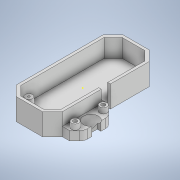
# Autodesk Inventor part: CameraMold
Saved by Autodesk Inventor 2020 (Build 240168000, 168)
## iProperties
Created: 2020-03-20
Part Number: CameraMold
Material: Generisch
Document SubType Name: Modeling
Designer: Fynn
Density: 1 g/cm^3
Appearance: Vorgabe
Author: Fynn
Autodesk Inventor part; units mm, degrees
ref_plane "YZ Plane" through (0, 0, 0) normal (1, 0, 0) x (0, 1, 0)
ref_plane "XZ Plane" through (0, 0, 0) normal (0, 1, 0) x (-1, 0, 0)
sketch "Skizze1" plane through (0, 0, 0) normal (0, 1, 0) x (-1, 0, 0)
  line L0 (-5.25, 27.5) -> (5.25, 27.5)
  line L1 (10.75, 22) -> (10.75, -22)
  line L2 (5.25, -27.5) -> (-5.25, -27.5)
  line L3 (-10.75, -22) -> (-10.75, 22)
  line L4 (-10.75, 27.5) -> (10.75, -27.5) construction
  line L5 (10.75, 27.5) -> (-10.75, -27.5) construction
  line L6 (10.75, 22) -> (5.25, 27.5)
  line L7 (10.75, -22) -> (5.25, -27.5)
  line L8 (-5.25, -27.5) -> (-10.75, -22)
  line L9 (-10.75, 22) -> (-5.25, 27.5)
  line L10 (7.25, 29.5) -> (-7.25, 29.5)
  line L11 (-12.75, 24) -> (-12.75, -24)
  line L12 (-7.25, -29.5) -> (7.25, -29.5)
  line L13 (12.75, -24) -> (12.75, 24)
  line L14 (12.75, 29.5) -> (-12.75, -29.5) construction
  line L15 (-12.75, 29.5) -> (12.75, -29.5) construction
  line L16 (12.75, 24) -> (7.25, 29.5)
  line L17 (12.75, -24) -> (7.25, -29.5)
  line L18 (-7.25, -29.5) -> (-12.75, -24)
  line L19 (-12.75, 24) -> (-7.25, 29.5)
  point P0 (0, 0)
  dimension "d0" = 21.5
  dimension "d1" = 55
  dimension "d2" = 5.5
  dimension "d3" = 5.5
  dimension "d4" = 5.5
  dimension "d5" = 5.5
  dimension "d6" = 5.5
  dimension "d7" = 5.5
  dimension "d8" = 5.5
  dimension "d9" = 5.5
  dimension "d10" = 2
  dimension "d11" = 2
  dimension "d12" = 5.5
  dimension "d13" = 5.5
  dimension "d14" = 5.5
  dimension "d15" = 5.5
  dimension "d16" = 5.5
  dimension "d17" = 5.5
  dimension "d18" = 5.5
  dimension "d19" = 5.5
  constraints: 40 end point, 16 point on line, 4 midpoint, 4 parallel, 2 horizontal, 2 perpendicular
  measures "d0" distance of L4.end L5.end
  measures "d1" distance of L5.start L4.end
  measures "d2" distance of L1.start L5.start
  measures "d3" distance of L0.end L5.start
  measures "d4" distance of L1.end L4.end
  measures "d5" distance of L2.start L4.end
  measures "d6" distance of L2.end L5.end
  measures "d7" distance of L3.start L5.end
  measures "d8" distance of L3.end L4.start
  measures "d9" distance of L0.start L4.start
  measures "d10" distance between parallel lines of L11 L3
  measures "d11" distance between parallel lines of L2 L12
  measures "d12" distance of L13.end L14.start
  measures "d13" distance of L10.start L14.start
  measures "d14" distance of L13.start L15.end
  measures "d15" distance of L12.end L15.end
  measures "d16" distance of L12.start L14.end
  measures "d17" distance of L11.end L14.end
  measures "d18" distance of L11.start L15.start
  measures "d19" distance of L10.end L15.start
extrude "Extrusion1" add sketch "Skizze1" along normal blind 10
sketch "Skizze3" plane through (0, 0, 0) normal (0, -1, 0) x (1, 0, 0)
  line L0 (7.25, -29.5) -> (-7.25, -29.5) projected
  line L1 (12.75, -24) -> (7.25, -29.5) projected
  line L2 (12.75, 24) -> (12.75, -24) projected
  line L3 (7.25, 29.5) -> (12.75, 24) projected
  line L4 (-7.25, 29.5) -> (7.25, 29.5) projected
  line L5 (-12.75, 24) -> (-7.25, 29.5) projected
  line L6 (-12.75, -24) -> (-12.75, 24) projected
  line L7 (-7.25, -29.5) -> (-12.75, -24) projected
  line L8 (-5.25, 27.5) -> (-10.75, 22) projected
  line L9 (5.25, 27.5) -> (-5.25, 27.5) projected
  line L10 (10.75, 22) -> (5.25, 27.5) projected
  line L11 (10.75, -22) -> (10.75, 22) projected
  line L12 (5.25, -27.5) -> (10.75, -22) projected
  line L13 (-5.25, -27.5) -> (5.25, -27.5) projected
  line L14 (-10.75, -22) -> (-5.25, -27.5) projected
  line L15 (-10.75, 22) -> (-10.75, -22) projected
  point P0 (0, 0)
extrude "Extrusion2" add sketch "Skizze3" along normal blind 2 contours L0 L7 L6 L5 L4 L3 L2 L1 | L9 L10 L11 L12 L13 L14 L15 L8
sketch "Skizze4" plane through (0, 0, 0) normal (0, 1, 0) x (1, 0, 0)
  line L0 (-10.75, -22) -> (-10.75, 22) projected
  line L1 (-10.75, -21) -> (-8.75, -21)
  line L2 (10.75, 22) -> (10.75, -22) projected
  line L3 (10.75, 18.3) -> (8.75, 18.3)
  circle A0 centre (-8.75, -21) radius 2
  circle A1 centre (8.75, 18.3) radius 2
  circle A2 centre (-8.75, -21) radius 0.55
  circle A3 centre (8.75, 18.3) radius 0.55
  point P0 (0, 0)
  dimension "d24" = 2
  dimension "d25" = 21
  dimension "d26" = 2
  dimension "d27" = 18.3
  dimension "d28" = 4
  dimension "d29" = 4
  dimension "d30" = 1.1
  dimension "d31" = 1.1
  constraints: 4 centre point, 4 coincident, 4 end point, 2 horizontal, 2 point on line
  measures "d24" distance of L1.start L1.end
  measures "d25" vertical distance of L1.start point (0, 0)
  measures "d26" distance of L3.start L3.end
  measures "d27" vertical distance of L3.start point (0, 0)
  measures "d28" diameter of A0
  measures "d29" diameter of A1
  measures "d30" diameter of A2
  measures "d31" diameter of A3
extrude "Extrusion3" add sketch "Skizze4" along normal blind 5
sketch "Skizze8" plane through (12.75, 10, 24) normal (1, 0, 0) x (0, 0, -1)
  line L0 (26.5, -23.1836) -> (21.5, -23.1836)
  line L1 (21.5, -23.1836) -> (21.5, 3.1836)
  line L2 (21.5, 3.1836) -> (26.5, 3.1836)
  line L3 (26.5, 3.1836) -> (26.5, -23.1836)
  line L4 (26.5, -23.1836) -> (21.5, 3.1836) construction
  line L5 (21.5, -23.1836) -> (26.5, 3.1836) construction
  point P0 (24, -10)
  dimension "d44" = 5
  constraints: 12 end point, 2 midpoint, 2 parallel, 1 horizontal, 1 perpendicular
  measures "d44" distance of L1.end L2.end
extrude "Extrusion7" cut sketch "Skizze8" against normal blind 8
sketch "Skizze9" plane through (0, -2, 0) normal (0, -1, 0) x (1, 0, 0)
  line L0 (4.75, -2.5) -> (4.75, 2.5) projected
  circle A0 centre (4.75, 0) radius 2.5
  point P0 (0, 0)
  point P1 (4.75, 2.5)
  constraints: 1 midpoint, 3 other
extrude "Extrusion8" cut sketch "Skizze9" against normal blind 12 contours A0 L0 picked at (4.3627, -0.7379)
sketch "Skizze17" plane through (0, 10, 0) normal (0, 1, 0) x (1, 0, 0)
  line L0 (6.25, -28) -> (-6.25, -28)
  line L1 (-11.25, -23) -> (-11.25, 23)
  line L2 (-6.25, 28) -> (6.25, 28)
  line L3 (11.25, 23) -> (11.25, -23)
  line L4 (11.25, -28) -> (-11.25, 28) construction
  line L5 (-11.25, -28) -> (11.25, 28) construction
  line L6 (-10.75, -22) -> (-10.75, 22) projected
  line L7 (5.25, -27.5) -> (-5.25, -27.5) projected
  line L8 (-11.25, -23) -> (-6.25, -28)
  line L9 (-11.25, 23) -> (-6.25, 28)
  line L10 (6.25, 28) -> (11.25, 23)
  line L11 (11.25, -23) -> (6.25, -28)
  line L12 (-5.25, -27.5) -> (-10.75, -22) projected
  line L13 (-10.75, 22) -> (-5.25, 27.5) projected
  line L14 (-5.25, 27.5) -> (5.25, 27.5) projected
  line L15 (5.25, 27.5) -> (10.75, 22) projected
  line L16 (10.75, 22) -> (10.75, 2.5) projected
  line L17 (10.75, -2.5) -> (10.75, -22) projected
  line L18 (10.75, -22) -> (5.25, -27.5) projected
  line L19 (12.75, -2.5) -> (10.75, -2.5) projected
  line L20 (10.75, -2.5) -> (10.75, 2.5)
  point P0 (0, 0)
  dimension "d74" = 0.5
  dimension "d75" = 0.5
  dimension "d80" = 5
  dimension "d81" = 5
  dimension "d82" = 5
  dimension "d83" = 5
  dimension "d84" = 5
  dimension "d85" = 5
  dimension "d86" = 5
  dimension "d87" = 5
  constraints: 22 end point, 12 point on line, 2 midpoint, 2 parallel, 2 perpendicular, 1 horizontal
  measures "d74" distance between parallel lines of L6 L1
  measures "d75" distance between parallel lines of L7 L0
  measures "d80" distance of L1.start point (-11.25, -28)
  measures "d81" distance of L0.end point (-11.25, -28)
  measures "d82" distance of L1.end L4.end
  measures "d83" distance of L2.start L4.end
  measures "d84" distance of L2.end L5.end
  measures "d85" distance of L3.start L5.end
  measures "d86" distance of L3.end L4.start
  measures "d87" distance of L0.start L4.start
extrude "Extrusion15" cut sketch "Skizze17" against normal up to surface (10 mm away)
sketch "Skizze18" plane through (12.75, -2, 24) normal (1, 0, 0) x (0, 0, -1)
  line L0 (21.5, 0) -> (21.5, 12) projected
  line L1 (0, 12) -> (21.5, 12) projected
  line L2 (0, 0) -> (0, 12) projected
  line L3 (21.5, 0) -> (0, 0) projected
  point P0 (24, 2)
extrude "Extrusion16" add sketch "Skizze18" along normal blind 10
ref_plane "Arbeitsebene1" through (0, 4, 0) normal (0, 1, 0) x (1, 0, 0)
sketch "Skizze19" plane through (0, 4, 0) normal (0, 1, 0) x (1, 0, 0)
  line L0 (12.75, -24) -> (7.25, -29.5) projected
  line L1 (4.75, -2.5) -> (22.75, -2.5) projected
  line L2 (12.75, -24) -> (22.75, -2.5)
  line L3 (22.75, -2.5) -> (22.75, -24) projected
  line L4 (22.75, -2.5) -> (22.75, -24)
  line L5 (22.75, -24) -> (12.75, -2.5)
  circle A0 centre (17.75, -13.25) radius 4.25
  line L6 (22, -13.25) -> (13.5, -13.25)
  point P0 (0, 0)
  dimension "d93" = 8.5
  constraints: 8 end point, 2 point on circle, 1 centre point, 1 collinear, 1 horizontal, 1 midpoint
  measures "d93" diameter of A0
revolve "Umdrehung1" cut sketch "Skizze19" angle 360 about axis through (22, 4, 13.25) along (-1, 0, 0) picked at (16.8466, -10.5822) picked at (14.953, -12.931) picked at (20.1235, -11.7363) contours A0 L2 L5 | L5 L6 A0 | A0 L6 L2
sketch "Skizze20" plane through (0, 10, 0) normal (0, 1, 0) x (1, 0, 0)
  line L0 (12.75, -24) -> (22.75, -24) projected
  line L1 (4.75, -2.5) -> (22.75, -2.5) projected
  line L2 (12.75, -24) -> (22.75, -2.5)
  line L3 (22.75, -2.5) -> (12.75, -2.5)
  line L4 (12.75, -24) -> (7.25, -29.5) projected
  line L5 (12.75, -24) -> (12.75, -2.5)
  line L6 (22.75, -2.5) -> (22.75, -24) projected
  point P0 (0, 0)
  constraints: 6 end point, 1 perpendicular, 1 point on line
extrude "Extrusion17" cut sketch "Skizze20" against normal blind 7
sketch "Skizze21" plane through (22.75, -2, 24) normal (1, 0, 0) x (0, 0, -1)
  line L0 (8.25, 12.4425) -> (13.25, 12.4425)
  line L1 (13.25, 12.4425) -> (13.25, -2.4425)
  line L2 (13.25, -2.4425) -> (8.25, -2.4425)
  line L3 (8.25, -2.4425) -> (8.25, 12.4425)
  line L4 (14.8807, 5) -> (6.6193, 5) projected
  line L5 (8.25, 12.4425) -> (13.25, -2.4425) construction
  line L6 (13.25, 12.4425) -> (8.25, -2.4425) construction
  point P0 (24, 2)
  point P1 (10.75, 5)
  point P2 (13.25, 5)
  point P3 (8.25, 5)
  dimension "d97" = 5
  constraints: 12 end point, 3 midpoint, 2 parallel, 1 horizontal, 1 perpendicular
  measures "d97" distance of L1.end L2.end
extrude "Extrusion18" cut sketch "Skizze21" against normal blind 4 contours L4 L1 L2 L3
sketch "Skizze22" plane through (22.75, -2, 24) normal (1, 0, 0) x (0, 0, -1)
  line L0 (-21.5, 10) -> (21.5, 10)
  line L1 (21.5, 10) -> (21.5, 0)
  line L2 (21.5, 0) -> (-21.5, 0)
  line L3 (-21.5, 0) -> (-21.5, 10)
  line L4 (-21.5, 10) -> (21.5, 0) construction
  line L5 (21.5, 10) -> (-21.5, 0) construction
  point P0 (24, 2)
  point P1 (0, 5)
  constraints: 12 end point, 2 midpoint, 2 parallel, 1 horizontal, 1 perpendicular
extrude "Extrusion19" cut sketch "Skizze22" against normal blind 2
sketch "Skizze23" plane through (0, 3, 0) normal (0, 1, 0) x (1, 0, 0)
  line L0 (20.75, -15.75) -> (20.75, -24) projected
  line L1 (12.75, -24) -> (12.75, -2.5) projected
  line L2 (20.75, -21) -> (16.75, -21)
  line L3 (16.75, -21) -> (16.75, -24)
  line L4 (12.75, -24) -> (20.75, -24) projected
  line L5 (20.75, -5.4005) -> (16.75, -5.4005)
  line L6 (16.75, -5.4005) -> (16.75, -2.4005)
  circle A0 centre (16.75, -21) radius 1.05
  circle A1 centre (16.75, -5.4005) radius 1.05
  point P0 (0, 0)
  dimension "d102" = 4
  dimension "d103" = 3
  dimension "d104" = 4
  dimension "d105" = 3
  dimension "d106" = 2.1
  dimension "d107" = 2.1
  constraints: 8 end point, 2 centre point, 2 coincident, 2 horizontal, 1 midpoint, 1 perpendicular, 1 point on line
  measures "d102" distance of L2.start L2.end
  measures "d103" distance of L2.end L3.end
  measures "d104" distance of L5.start L5.end
  measures "d105" distance of L5.end L6.end
  measures "d106" diameter of A0
  measures "d107" diameter of A1
extrude "Extrusion20" cut sketch "Skizze23" against normal through all contours A0 L3 L2 | L2 L3 A0 | A1 L6 L5 | L5 L6 A1
sketch "Skizze24" plane through (0, 3, 0) normal (0, 1, 0) x (1, 0, 0)
  point P0 (0, 0)
sketch "Skizze25" plane through (0, 3, 0) normal (0, 1, 0) x (1, 0, 0)
  circle A0 centre (16.75, -5.4005) radius 1.05 projected
  circle A1 centre (16.75, -5.4005) radius 2
  circle A2 centre (16.75, -21) radius 1.05 projected
  circle A3 centre (16.75, -21) radius 2
  point P0 (0, 0)
  dimension "d110" = 4
  dimension "d111" = 4
  constraints: 2 centre point, 2 coincident
  measures "d110" diameter of A1
  measures "d111" diameter of A3
extrude "Extrusion21" add sketch "Skizze25" along normal blind 3
sketch "Skizze26" plane through (0, 3, 0) normal (0, 1, 0) x (1, 0, 0)
  point P0 (0, 0)
chamfer "Fase2" distance 4 angle 45 2 edges at (20.75, 0.5, 2.5) (20.75, 0.5, 24)
fillet "Rundung2" radius 4 2 edges at (20.75, 0.5, 20) (20.75, 0.5, 6.5)
equation "\"d3\" = d2"
equation "\"d5\" = d4"
equation "\"d6\" = d4"
equation "\"d7\" = d6"
equation "\"d8\" = d4"
equation "\"d9\" = d8"
equation "\"d13\" = d12"
equation "\"d14\" = d12"
equation "\"d15\" = d14"
equation "\"d16\" = d12"
equation "\"d17\" = d16"
equation "\"d18\" = d12"
equation "\"d19\" = d18"
equation "\"d81\" = d80"
equation "\"d83\" = d82"
equation "\"d84\" = d82"
equation "\"d85\" = d84"
equation "\"d86\" = d82"
equation "\"d87\" = d86"
